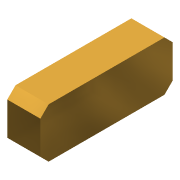
# Autodesk Inventor part: Key
Saved by Autodesk Inventor 2022 Beta2 (Build 260130000, 130) ContinuousBuild 0
## iProperties
Shininess: 64.0
Angle Display Precision: 2
Document Length Units: 11272
Document Angle Units: 11279
Document Time Units: 11290
Document Mass Units: 11286
Document Length Units Precision: 3
Document Angle Units Precision: 2
Created: 2002-04-23
Part Number: Key
Material: Brass, Soft Yellow
Document SubType Name: Modeling
Designer: Nino
Density: 8.47 g/cm^3
Mass: 101.93 g
Surface Area: 35.7487 cm^2
Volume: 12.0343 cm^3
Appearance: Brass - Satin
Density: 0.0
Volumn: 0.0
Area: 0.0
PropertySet Name: Model Information
Control State: 0
Master: False
Checked Out: False
Author: Nino
Autodesk Inventor part; units mm, degrees
ref_plane "YZ Plane" through (0, 0, 0) normal (1, 0, 0) x (0, 1, 0)
ref_plane "XZ Plane" through (0, 0, 0) normal (0, 1, 0) x (-1, 0, 0)
ref_plane "XY Plane" through (0, 0, 0) normal (0, 0, 1) x (1, 0, 0)
sketch "Sketch1" plane through (0, 0, 0) normal (0, 0, 1) x (1, 0, 0)
  line L0 (-16.3539, 20.2564) -> (-3.6539, 20.2564)
  line L1 (-3.6539, 20.2564) -> (-3.6539, 1.2064)
  line L2 (-3.6539, 1.2064) -> (-16.3539, 1.2064)
  line L3 (-16.3539, 1.2064) -> (-16.3539, 20.2564)
  dimension "d0" = 12.7
  dimension "d1" = 19.05
  constraints: 8 end point, 2 parallel, 1 horizontal, 1 perpendicular
  measures "d0" distance between parallel lines of L1 L3
  measures "d1" distance between parallel lines of L0 L2
extrude "Extrusion1" add sketch "Sketch1" along normal blind 50.8
chamfer "Chamfer1" distance 3.175 angle 45 4 edges at (-10.0039, 20.2564, 50.8) (-10.0039, 20.2564, 0) (-10.0039, 1.2064, 50.8) (-10.0039, 1.2064, 0)
equation "\"d1\" = 1.5 * d0"
body "Solid1"
